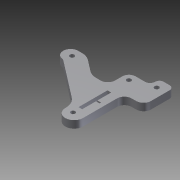
# Autodesk Inventor part: braket bawah
Saved by Autodesk Inventor 2012 (Build 160160000, 160)
## iProperties
Created: 2013-12-07
Part Number: braket bawah
Material: Default
Document SubType Name: Modeling
Designer: Irwan Haryanto
Density: 1 g/cm^3
Author: Irwan Haryanto
Autodesk Inventor part; units mm, degrees
ref_plane "YZ Plane" through (0, 0, 0) normal (1, 0, 0) x (0, 1, 0)
ref_plane "XZ Plane" through (0, 0, 0) normal (0, 1, 0) x (-1, 0, 0)
ref_plane "XY Plane" through (0, 0, 0) normal (0, 0, 1) x (1, 0, 0)
sketch "Sketch1" plane through (0, 0, 0) normal (0, 0, 1) x (1, 0, 0)
  line L0 (17.4112, 0) -> (20.3, 0)
  line L1 (29.8, -3.5) -> (31.05, -3.5)
  line L2 (31.05, -23.3) -> (28.55, -23.3)
  line L3 (28.55, -23.3) -> (28.55, -3.5)
  line L4 (28.55, -3.5) -> (29.8, -3.5)
  line L5 (29.8, -23.3) -> (29.8, -28.3)
  line L6 (31.05, -23.3) -> (31.05, -13.9)
  line L7 (31.05, -13.9) -> (33.55, -13.9)
  line L8 (33.55, -13.9) -> (33.55, -12.9)
  line L9 (33.55, -12.9) -> (31.05, -12.9)
  line L10 (31.05, -12.9) -> (31.05, -3.5)
  line L11 (36.55, -14.9) -> (36.55, -28.3)
  line L12 (49.7, 17.8) -> (49.7, 5)
  line L13 (36.55, -13) -> (36.55, -14.9)
  arc A0 (24.55, -28.3) -> (36.55, -28.3) centre (30.55, -28.3) ccw
  line L14 (24.55, -27.924) -> (24.55, -28.3)
  line L15 (5.8588, -8.6221) -> (20.6471, -19.9978)
  arc A1 (29.8, 14.4) -> (25.3, 9.9) centre (29.8, 9.9) ccw
  line L16 (25.3, 9.9) -> (25.3, 5)
  line L17 (36.55, -13) -> (36.55, -5)
  line L18 (44.7, 0) -> (41.55, 0)
  line L19 (36.3, 14.4) -> (29.8, 14.4)
  arc A2 (36.3, 14.4) -> (39.7, 17.8) centre (36.3, 17.8) ccw
  arc A3 (41.55, 0) -> (36.55, -5) centre (41.55, -5) ccw
  arc A4 (44.7, 0) -> (49.7, 5) centre (44.7, 5) ccw
  arc A5 (20.3, 0) -> (25.3, 5) centre (20.3, 5) ccw
  arc A6 (24.55, -27.924) -> (20.6471, -19.9978) centre (14.55, -27.924) ccw
  line L20 (-3.96, 9.9) -> (-2.2612, 9.9)
  line L21 (-3.96, 9.9) -> (-5, 9.9)
  line L22 (-10, 4.9) -> (-10, 4.7)
  line L23 (11.3141, 2.0738) -> (3.8359, 7.8262)
  arc A7 (11.3141, 2.0738) -> (17.4112, 0) centre (17.4112, 10) ccw
  arc A8 (3.8359, 7.8262) -> (-2.2612, 9.9) centre (-2.2612, -0.1) ccw
  arc A9 (-5, 9.9) -> (-10, 4.9) centre (-5, 4.9) ccw
  arc A10 (-10, 4.7) -> (-5.7001, -0.2507) centre (-5, 4.7) ccw
  line L24 (5.8588, -8.6221) -> (-4.2953, -0.8401)
  arc A11 (-4.2953, -0.8401) -> (-5.7001, -0.2507) centre (-6.1202, -3.2212) ccw
  line L25 (39.7, 17.8) -> (39.7, 17.8)
  line L26 (49.7, 17.8) -> (49.7, 17.8)
  line L27 (44.7, 20.8) -> (46.7, 20.8)
  line L28 (44.7, 20.8) -> (42.7, 20.8)
  arc A12 (42.7, 20.8) -> (39.7, 17.8) centre (42.7, 17.8) ccw
  arc A13 (49.7, 17.8) -> (46.7, 20.8) centre (46.7, 17.8) ccw
  point P0 (0, 0)
  dimension "d0" = 1.25
  dimension "d1" = 2.5
  dimension "d2" = 19.8
  dimension "d3" = 5
  dimension "d4" = 9.4
  dimension "d5" = 2.5
  dimension "d6" = 1
  dimension "d7" = 5
  dimension "d8" = 5
  dimension "d9" = 10
  dimension "d10" = 10
  dimension "d11" = 5
  dimension "d12" = 3
  dimension "d13" = 3
  constraints: 58 end point, 28 point on circle, 21 tangent, 14 centre point, 4 equal radius, 1 midpoint, 1 perpendicular, 1 point on line
  measures "d0" distance of L1.start L1.end
  measures "d1" distance of L2.start L2.end
  measures "d2" distance of L2.end L3.end
  measures "d3" distance of L5.start L5.end
  measures "d4" distance of L2.start L6.end
  measures "d5" distance of L6.end L7.end
  measures "d6" distance of L7.end L8.end
  measures "d7" radius of A3
  measures "d8" radius of A5
  measures "d9" radius of A6
  measures "d10" radius of A7
  measures "d11" radius of A9
  measures "d12" radius of A11
  measures "d13" radius of A12
extrude "Extrusion1" add sketch "Sketch1" along normal blind 5
sketch "Sketch2" plane through (0, 0, 5) normal (0, 0, 1) x (1, 0, 0)
  arc A0 (29.8, 14.4) -> (25.3, 9.9) centre (29.8, 9.9) ccw projected
  line L0 (17.4112, 0) -> (20.3, 0)
  circle A1 centre (43.66, 15) radius 1.5
  circle A2 centre (-3.96, 4.8) radius 1.5
  line L1 (29.8, -3.5) -> (31.05, -3.5)
  line L2 (31.05, -23.3) -> (28.55, -23.3)
  line L3 (28.55, -23.3) -> (28.55, -3.5)
  line L4 (28.55, -3.5) -> (29.8, -3.5)
  line L5 (29.8, -23.3) -> (29.8, -28.3)
  circle A3 centre (29.8, -28.3) radius 1.5
  line L6 (31.05, -23.3) -> (31.05, -13.9)
  line L7 (31.05, -13.9) -> (33.55, -13.9)
  line L8 (33.55, -13.9) -> (33.55, -12.9)
  line L9 (33.55, -12.9) -> (31.05, -12.9)
  line L10 (31.05, -12.9) -> (31.05, -3.5)
  line L11 (36.55, -14.9) -> (36.55, -28.3)
  line L12 (49.7, 17.8) -> (49.7, 5)
  line L13 (36.55, -13) -> (36.55, -14.9)
  arc A4 (24.55, -28.3) -> (36.55, -28.3) centre (30.55, -28.3) ccw
  line L14 (24.55, -27.924) -> (24.55, -28.3)
  line L15 (5.8588, -8.6221) -> (20.6471, -19.9978)
  circle A5 centre (29.8, 9.9) radius 1.5
  arc A6 (29.8, 14.4) -> (25.3, 9.9) centre (29.8, 9.9) ccw
  line L16 (25.3, 9.9) -> (25.3, 5)
  line L17 (36.55, -13) -> (36.55, -5)
  line L18 (44.7, 0) -> (41.55, 0)
  line L19 (36.3, 14.4) -> (29.8, 14.4)
  arc A7 (36.3, 14.4) -> (39.7, 17.8) centre (36.3, 17.8) ccw
  arc A8 (41.55, 0) -> (36.55, -5) centre (41.55, -5) ccw
  arc A9 (44.7, 0) -> (49.7, 5) centre (44.7, 5) ccw
  arc A10 (20.3, 0) -> (25.3, 5) centre (20.3, 5) ccw
  arc A11 (24.55, -27.924) -> (20.6471, -19.9978) centre (14.55, -27.924) ccw
  line L20 (-3.96, 9.9) -> (-2.2612, 9.9)
  line L21 (-3.96, 9.9) -> (-5, 9.9)
  line L22 (-10, 4.9) -> (-10, 4.7)
  line L23 (11.3141, 2.0738) -> (3.8359, 7.8262)
  arc A12 (11.3141, 2.0738) -> (17.4112, 0) centre (17.4112, 10) ccw
  arc A13 (3.8359, 7.8262) -> (-2.2612, 9.9) centre (-2.2612, -0.1) ccw
  arc A14 (-5, 9.9) -> (-10, 4.9) centre (-5, 4.9) ccw
  arc A15 (-10, 4.7) -> (-5.7001, -0.2507) centre (-5, 4.7) ccw
  line L24 (5.8588, -8.6221) -> (-4.2953, -0.8401)
  arc A16 (-4.2953, -0.8401) -> (-5.7001, -0.2507) centre (-6.1202, -3.2212) ccw
  line L25 (39.7, 17.8) -> (39.7, 17.8)
  line L26 (49.7, 17.8) -> (49.7, 17.8)
  line L27 (44.7, 20.8) -> (46.7, 20.8)
  line L28 (44.7, 20.8) -> (42.7, 20.8)
  arc A17 (42.7, 20.8) -> (39.7, 17.8) centre (42.7, 17.8) ccw
  arc A18 (49.7, 17.8) -> (46.7, 20.8) centre (46.7, 17.8) ccw
  point P0 (0, 0)
  dimension "d16" = 1.25
  dimension "d17" = 2.5
  dimension "d18" = 19.8
  dimension "d19" = 5
  dimension "d20" = 9.4
  dimension "d21" = 2.5
  dimension "d22" = 1
  dimension "d23" = 5
  dimension "d24" = 5
  dimension "d25" = 10
  dimension "d26" = 10
  dimension "d27" = 5
  dimension "d28" = 3
  dimension "d29" = 3
  constraints: 58 end point, 28 point on circle, 21 tangent, 18 centre point, 4 equal radius, 2 coincident, 1 midpoint, 1 perpendicular, 1 point on line
  measures "d16" distance of L1.start L1.end
  measures "d17" distance of L2.start L2.end
  measures "d18" distance of L2.end L3.end
  measures "d19" distance of L5.start L5.end
  measures "d20" distance of L2.start L6.end
  measures "d21" distance of L6.end L7.end
  measures "d22" distance of L7.end L8.end
  measures "d23" radius of A8
  measures "d24" radius of A10
  measures "d25" radius of A11
  measures "d26" radius of A12
  measures "d27" radius of A14
  measures "d28" radius of A16
  measures "d29" radius of A17
hole "Hole1" at (29.8, -28.3, 5) at (43.66, 15, 5) at (29.8, 9.9, 5) at (-3.96, 4.8, 5) direction (0, 0, -1) diameter 3 end through all
body "Solid1"
